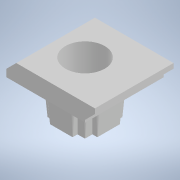
# Autodesk Inventor part: wm_one_door_lock_na
Saved by Autodesk Inventor 2021 (Build 250183000, 183)
## iProperties
Created: 2025-08-10
Part Number: wm_one_door_lock_na
Material: Generic
Catalog Web Link: www.cadenas.de
Description: WM ONE DOOR LOCK-WALLMOUNT
Vendor: RITTAL
Document SubType Name: Modeling
Designer: psAdmin
Manufacturer: RITTAL
Mass: 8.51227 g
Surface Area: 49.1686 cm^2
Volume: 8.51227 cm^3
Density: 1 g/cm^3
Appearance: PSOLRGB-175-175-175
Category: PARTsolutions
Company: RITTAL
Title: wm_one_door_lock_na
Author: Cadenas PARTsolutions
Comments: WALLMOUNT
PSOL_IDENT_0: {$CADENAS_DATA/23d-libs/rittal/rittal_north_america/enclosure_systems/compact_enclosures/wm_parts/wm
PSOL_IDENT_1: _one_door_parts/lock.prj},188 {VTYP=3D},{NB=wm_one_door_lock_na},{LINA=wm_one_door_lock_na},{NN=WM O
PSOL_IDENT_2: NE DOOR LOCK},{DATE=20.08.2024 09:24:21},{GEOMDATE=25.11.2019 11:27:46},{VERSION=},{LINEID=10},{WBVA
PSOL_IDENT_3: R=},{WBNUMERIC=}  {NB=wm_one_door_lock_na},{LINA=wm_one_door_lock_na},{KT=DUMMY},{PN=wm_one_door_loc
PSOL_IDENT_4: k},{DETAIL=MIN}
NB: wm_one_door_lock_na
NN: WM ONE DOOR LOCK
NT: WALLMOUNT
NBSYN: $PN._na
LINA: wm_one_door_lock_na
CATALOG: Rittal
PN: wm_one_door_lock
DETAIL: 0
SUPPLIER: RITTAL
ARTICLENO: wm_one_door_lock_na
BOMINFO: wm_one_door_lock_na
CREATOR: CADENAS GmbH
Autodesk Inventor part; units mm, degrees
sketch "Sketch_1" plane through (0, 0, 0) normal (0, 0, 1) x (1, 0, 0)
  line L0 (-18, -4) -> (14, -4)
  line L1 (14, -4) -> (14, -3)
  line L2 (14, -3) -> (18, 1)
  line L3 (18, 1) -> (18, 3)
  line L4 (18, 3) -> (-14, 3)
  line L5 (-14, 3) -> (-18, -1)
  line L6 (-18, -1) -> (-18, -4)
  constraints: 14 end point
extrude "Extrusion1" add sketch "Sketch_1" along normal mid plane 32
sketch "Sketch_2" plane through (0, -3, 0) normal (0, 1, 0) x (1, 0, 0)
  arc A0 (-13.055, -4.46) -> (-11.555, -5.96) centre (-11.555, -4.46) ccw
  line L0 (-11.555, -5.96) -> (-11.045, -5.96)
  line L1 (-11.045, -5.96) -> (-11.045, -7.49)
  arc A1 (-11.045, -7.49) -> (-9.545, -8.99) centre (-9.545, -7.49) ccw
  line L2 (-9.545, -8.99) -> (-8.015, -8.99)
  line L3 (-8.015, -8.99) -> (-8.015, -9.5)
  arc A2 (-8.015, -9.5) -> (-6.515, -11) centre (-6.515, -9.5) ccw
  line L4 (-6.515, -11) -> (2.405, -11)
  arc A3 (2.405, -11) -> (3.905, -9.5) centre (2.405, -9.5) ccw
  line L5 (3.905, -9.5) -> (3.905, -8.99)
  line L6 (3.905, -8.99) -> (5.435, -8.99)
  arc A4 (5.435, -8.99) -> (6.935, -7.49) centre (5.435, -7.49) ccw
  line L7 (6.935, -7.49) -> (6.935, -5.96)
  line L8 (6.935, -5.96) -> (7.445, -5.96)
  arc A5 (7.445, -5.96) -> (8.945, -4.46) centre (7.445, -4.46) ccw
  line L9 (8.945, -4.46) -> (8.945, 4.46)
  arc A6 (8.945, 4.46) -> (7.445, 5.96) centre (7.445, 4.46) ccw
  line L10 (7.445, 5.96) -> (6.935, 5.96)
  line L11 (6.935, 5.96) -> (6.935, 7.49)
  arc A7 (6.935, 7.49) -> (5.435, 8.99) centre (5.435, 7.49) ccw
  line L12 (5.435, 8.99) -> (3.905, 8.99)
  line L13 (3.905, 8.99) -> (3.905, 9.5)
  arc A8 (3.905, 9.5) -> (2.405, 11) centre (2.405, 9.5) ccw
  line L14 (2.405, 11) -> (-6.515, 11)
  arc A9 (-6.515, 11) -> (-8.015, 9.5) centre (-6.515, 9.5) ccw
  line L15 (-8.015, 9.5) -> (-8.015, 8.99)
  line L16 (-8.015, 8.99) -> (-9.545, 8.99)
  arc A10 (-9.545, 8.99) -> (-11.045, 7.49) centre (-9.545, 7.49) ccw
  line L17 (-11.045, 7.49) -> (-11.045, 5.96)
  line L18 (-11.045, 5.96) -> (-11.555, 5.96)
  arc A11 (-11.555, 5.96) -> (-13.055, 4.46) centre (-11.555, 4.46) ccw
  line L19 (-13.055, 4.46) -> (-13.055, -4.46)
  constraints: 40 end point, 24 point on circle, 12 centre point
extrude "Extrusion2" add sketch "Sketch_2" against normal blind 15 draft -5
sketch "Sketch3" plane through (-14, 3, 16) normal (0, 1, 0) x (1, 0, 0)
  point P0 (12, 16)
hole "Hole1" at (-2, 3, 0) direction (0, -1, 0) diameter 10.2 depth 21 counterbore diameter 16 counterbore depth 18.5
ref_plane "insrt_to_lock_XY" through (-2, 3, 0) normal (0, 1, 0) x (1, 0, 0)
ref_plane "insrt_to_lock_YZ" through (-2, 3, 0) normal (1, 0, 0) x (0, 0, -1)
ref_plane "insrt_to_lock_ZX" through (-2, 3, 0) normal (0, 0, -1) x (0, 1, 0)
ref_plane "lock_to_body_XY" through (0, 3, 0) normal (0, 1, 0) x (1, 0, 0)
ref_plane "lock_to_body_YZ" through (0, 3, 0) normal (1, 0, 0) x (0, 0, -1)
ref_plane "lock_to_body_ZX" through (0, 3, 0) normal (0, 0, -1) x (0, 1, 0)
ref_plane "washer_XY" through (-2, -18.5, 0) normal (0, 1, 0) x (1, 0, 0)
ref_plane "washer_YZ" through (-2, -18.5, 0) normal (1, 0, 0) x (0, 0, -1)
ref_plane "washer_ZX" through (-2, -18.5, 0) normal (0, 0, -1) x (0, 1, 0)
body "Solid1"
